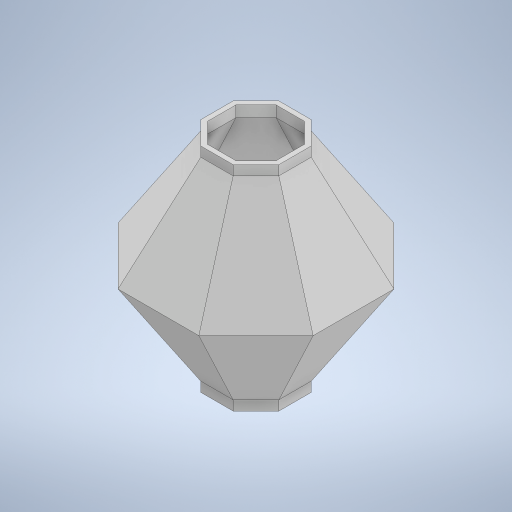
# Autodesk Inventor part: OV-PAM_tendon
Saved by Autodesk Inventor 2024 (Build 280153000, 153)
## iProperties
Created: 2023-07-13
Part Number: OV-PAM_tendon
Material: 일반
Document SubType Name: Modeling
Designer: jsw
Density: 1 g/cm^3
Appearance: 기본값
Author: jsw
Autodesk Inventor part; units mm, degrees
ref_plane "YZ Plane" through (0, 0, 0) normal (1, 0, 0) x (0, 1, 0)
sketch "스케치1" plane through (0, 0, 0) normal (0, 1, 0) x (-1, 0, 0)
  line L0 (12.0711, -5) -> (5, -12.0711)
  line L1 (5, -12.0711) -> (-5, -12.0711)
  line L2 (-5, -12.0711) -> (-12.0711, -5)
  line L3 (-12.0711, -5) -> (-12.0711, 5)
  line L4 (-12.0711, 5) -> (-5, 12.0711)
  line L5 (-5, 12.0711) -> (5, 12.0711)
  line L6 (5, 12.0711) -> (12.0711, 5)
  line L7 (12.0711, 5) -> (12.0711, -5)
  point P0 (0, 0)
  point P1 (0, 0)
  dimension "d0" = 10
  constraints: 16 end point, 1 coincident, 1 horizontal, 17 other
  measures "d0" distance of L6.end L0.start
extrude "돌출1" add sketch "스케치1" along normal blind 12
sketch "스케치3" plane through (0, 12, 0) normal (0, 1, 0) x (1, 0, 0)
  line L0 (2, -4.8284) -> (-2, -4.8284)
  line L1 (-2, -4.8284) -> (-4.8284, -2)
  line L2 (-4.8284, -2) -> (-4.8284, 2)
  line L3 (-4.8284, 2) -> (-2, 4.8284)
  line L4 (-2, 4.8284) -> (2, 4.8284)
  line L5 (2, 4.8284) -> (4.8284, 2)
  line L6 (4.8284, 2) -> (4.8284, -2)
  line L7 (4.8284, -2) -> (2, -4.8284)
  line L8 (5, 12.0711) -> (-5, 12.0711) projected
  line L9 (0, 0) -> (5, 12.0711)
  line L10 (5, 12.0711) -> (-5, 12.0711)
  line L11 (-5, 12.0711) -> (0, 0)
  dimension "d5" = 4
  constraints: 22 end point, 1 coincident, 1 collinear, 1 horizontal, 17 other
  measures "d5" distance of L0.start L0.end
ref_plane "작업 평면3" through (5, 0, -12.0711) normal (0, 0.5167309, -0.8561478) x (-1, 0, 0)
sketch "스케치4" plane through (5, 0, -12.0711) normal (0, 0, -1) x (-1, 0, 0)
  line L0 (0, 0) -> (0, 12) projected
  line L1 (10, 0) -> (0, 0) projected
  line L2 (0, 12) -> (0, 0)
  line L3 (0, 0) -> (10, 0)
  line L4 (10, 12) -> (0, 12) projected
  line L5 (10, 0) -> (10, 12)
  line L6 (10, 12) -> (0, 12)
  point P0 (5, 0)
  constraints: 8 end point, 3 perpendicular, 1 collinear
extrude "돌출2" cut sketch "스케치4" along normal up to surface surface through (5, 0, -12.0711) normal (0, 0.5167309, -0.8561478)
pattern_circular "원형 패턴1" count 8 over 360 about axis through (0, -10, 0) along (0, 1, 0) of "돌출2"
ref_plane "작업 평면4" through (0, 0, 0) normal (0, -1, 0) x (1, 0, 0)
sketch "스케치5" plane through (0, 12, 0) normal (0, 1, 0) x (1, 0, 0)
  line L0 (4.8284, 2) -> (2, 4.8284) projected
  line L1 (2, 4.8284) -> (-2, 4.8284) projected
  line L2 (-2, 4.8284) -> (-4.8284, 2) projected
  line L3 (-4.8284, 2) -> (-4.8284, -2) projected
  line L4 (-4.8284, -2) -> (-2, -4.8284) projected
  line L5 (-2, -4.8284) -> (2, -4.8284) projected
  line L6 (2, -4.8284) -> (4.8284, -2) projected
  line L7 (4.8284, -2) -> (4.8284, 2) projected
  point P0 (0, 0)
extrude "돌출3" add sketch "스케치5" along normal blind 1.2
mirror "미러1" about plane through (0, 0, 0) normal (0, -1, 0) of "돌출2", "원형 패턴1", "돌출3", "돌출1"
shell "쉘1" thickness 0.6 removed faces 2 at (-0.6667, 13.2, -1.6095) at (-0.6667, -13.2, -1.6095)
